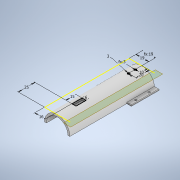
# Autodesk Inventor part: smart_pen4
Saved by Autodesk Inventor 2020 (Build 240168000, 168)
## iProperties
Created: 2022-09-28
Part Number: smart_pen4
Material: 일반
Document SubType Name: Modeling
Designer: taewo
Density: 1 g/cm^3
Appearance: 기본값
Author: taewo
Autodesk Inventor part; units mm, degrees
ref_plane "YZ Plane" through (0, 0, 0) normal (1, 0, 0) x (0, 1, 0)
ref_plane "XZ Plane" through (0, 0, 0) normal (0, 1, 0) x (-1, 0, 0)
ref_plane "XY Plane" through (0, 0, 0) normal (0, 0, 1) x (1, 0, 0)
sketch "roof_sketch" plane through (0, 0, 0) normal (0, 0, 1) x (1, 0, 0)
  line L0 (-26.6, 0) -> (26.6, 0) construction
  line L1 (0, -3.8) -> (0, 22.8) construction
  line L2 (-16, 0) -> (16, 0)
  line L3 (-19, 0) -> (-16, 0)
  line L4 (16, 0) -> (19, 0)
  arc A0 (16, 0) -> (-16, 0) centre (0, 0) ccw
  arc A1 (19, 0) -> (-19, 0) centre (0, 0) ccw
  line L5 (-19, 0) -> (-16, 0)
  line L6 (16, 0) -> (19, 0)
  dimension "d1" = 32
  dimension "d5" = 0
  dimension "d6" = 3
  constraints: 10 end point, 4 point on circle, 2 centre point, 2 collinear, 2 horizontal, 1 coincident, 1 point on line
  measures "d1" distance of L2.start L2.end
  measures "d5" distance between parallel lines of L0 L2
  measures "d6" radial gap between concentric circles of A1 A0
extrude "roof" add sketch "roof_sketch" along normal blind 126.5 contours L3 A1 L4 A0
sketch "bolt_sketch" plane through (16, 0, 0) normal (0, -1, 0) x (1, 0, 0)
  line L0 (-52.4, 0) -> (20.4, 0) construction
  line L1 (-16, -25.3) -> (-16, 151.8) construction
  line L2 (3, 0) -> (3, 126.5) projected
  line L3 (3, 41.5) -> (10, 41.5)
  line L4 (10, 41.5) -> (10, 0)
  line L5 (10, 0) -> (3, 0)
  line L6 (3, 0) -> (3, 41.5)
  circle A0 centre (6.5, 31.5) radius 1.5
  circle A1 centre (6.5, 11.5) radius 1.5
  line L7 (-35, 41.5) -> (-42, 41.5)
  line L8 (-42, 41.5) -> (-42, 0)
  line L9 (-42, 0) -> (-35, 0)
  line L10 (-35, 0) -> (-35, 41.5)
  circle A2 centre (-38.5, 31.5) radius 1.5
  circle A3 centre (-38.5, 11.5) radius 1.5
  point P0 (-16, 0)
  dimension "d9" = 41.5
  dimension "d10" = 3
  dimension "d11" = 3
  dimension "d12" = 10
  dimension "d13" = 20
  dimension "d14" = 7
  dimension "d16" = 3.5
  dimension "d17" = 3.5
  constraints: 16 end point, 7 symmetric about line, 4 centre point, 2 parallel, 2 point on line, 1 horizontal, 1 perpendicular, 2 other
  measures "d9" distance of L3.end L4.end
  measures "d10" diameter of A0
  measures "d11" diameter of A1
  measures "d12" distance from line of L3 A0.centre
  measures "d13" distance of A1.centre A0.centre
  measures "d14" distance of L3.start L3.end
  measures "d16" distance from line of L4 A0.centre
  measures "d17" distance from line of L4 A1.centre
extrude "bolt_opposite" add sketch "bolt_sketch" against normal blind 1.5
sketch "error1_" plane through (-19, 0, 0) normal (1, 0, 0) x (0, 0, -1)
  line L0 (0, 1.5) -> (-41.5, 1.5) projected
  line L1 (0, 0) -> (0, 1.5) projected
  line L2 (-41.5, 0) -> (0, 0) projected
  line L3 (-41.5, 0) -> (-41.5, 1.5) projected
extrude "error1" add sketch "error1_" along normal blind 1.5
sketch "error2_" plane through (19, 0, 0) normal (-1, 0, 0) x (0, 0, 1)
  line L0 (0, 0) -> (0, 1.5) projected
  line L1 (0, 1.5) -> (41.5, 1.5) projected
  line L2 (41.5, 0) -> (0, 0) projected
  line L3 (41.5, 0) -> (41.5, 1.5) projected
extrude "error2" add sketch "error2_" along normal blind 1.5
ref_plane "for_button" through (16, 19, 126.5) normal (0, -1, 0) x (1, 0, 0)
sketch "button_sketch" plane through (16, 19, 126.5) normal (0, -1, 0) x (1, 0, 0)
  line L0 (-13, -25) -> (-19, -25)
  line L1 (-19, -25) -> (-19, -40)
  line L2 (-19, -40) -> (-13, -40)
  line L3 (-13, -40) -> (-13, -25)
  line L4 (-35, -85) -> (-35, 0) projected
  line L5 (3, 0) -> (-35, 0) projected
  circle A0 centre (-15.9407, -106.5001) radius 1.5
  circle A1 centre (-15.9407, -116.5) radius 1.5
  line L6 (2.9407, -126.5) -> (-34.9407, -126.5) projected
  line L7 (-34.9407, -126.5) -> (-34.9407, -85) projected
  point P0 (-16, -126.5)
  dimension "d25" = 6
  dimension "d26" = 15
  dimension "d27" = 16
  dimension "d28" = 25
  dimension "d43" = 3
  dimension "d44" = 3
  dimension "d45" = 10
  dimension "d46" = 20
  dimension "d47" = 19
  dimension "d48" = 19
  constraints: 8 end point, 2 centre point, 2 parallel, 1 horizontal, 1 perpendicular
  measures "d25" distance of L1.end L2.end
  measures "d26" distance of L0.end L1.end
  measures "d27" distance between parallel lines of L4 L1
  measures "d28" distance between parallel lines of L5 L0
  measures "d43" diameter of A0
  measures "d44" diameter of A1
  measures "d45" distance from line of L6 A1.centre
  measures "d46" distance of point (-16, -126.5) A0.centre
  measures "d47" distance from line of L7 A0.centre
  measures "d48" distance from line of L7 A1.centre
extrude "button" cut sketch "button_sketch" along normal blind 10 contours L3 L2 L1 L0
fillet "so_hurt" radius 0.7 4 edges at (26, 1.5, 20.75) (22.4703, 1.5, 41.5) (-26, 1.5, 20.75) (-22.4703, 1.5, 41.5)
extrude "bar" cut sketch "button_sketch" along normal blind 10 contours A0 | A1
equation "\"d11\" = d10"
equation "\"d16\" = 0.5 * d14"
equation "\"d17\" = d16"
equation "\"d44\" = d43"
equation "\"d48\" = d47"
